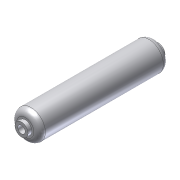
# Autodesk Inventor part: Pneuare Tank
Saved by Autodesk Inventor 2012 (Build 160160000, 160)
## iProperties
Created: 2013-02-02
Part Number: Pneuare Tank
Material: Polypropylene
Document SubType Name: Modeling
Designer: JesseK
Density: 0.899 g/cm^3
Mass: 311.75 g
Surface Area: 1100.4 cm^2
Volume: 346.774 cm^3
Author: JesseK
Autodesk Inventor part; units mm, degrees
ref_plane "YZ Plane" through (0, 0, 0) normal (1, 0, 0) x (0, 1, 0)
ref_plane "XZ Plane" through (0, 0, 0) normal (0, 1, 0) x (-1, 0, 0)
ref_plane "XY Plane" through (0, 0, 0) normal (0, 0, 1) x (1, 0, 0)
sketch "Sketch1" plane through (0, 0, 0) normal (0, 0, 1) x (1, 0, 0)
  circle A0 centre (0, 0) radius 31.75
  dimension "d0" = 63.5
  constraints: 1 centre point, 1 coincident
  measures "d0" diameter of A0
extrude "Extrusion1" add sketch "Sketch1" along normal blind 286.0294
sketch "Sketch2" plane through (0, 0, 286.0294) normal (0, 0, 1) x (1, 0, 0)
  circle A0 centre (0, 0) radius 31.75 projected
  circle A1 centre (0, 0) radius 14.5034
  dimension "d3" = 29.0068
  constraints: 1 centre point, 1 coincident
  measures "d3" diameter of A1
extrude "Extrusion2" add sketch "Sketch2" along normal blind 8.3566 contours A1
sketch "Sketch3" plane through (0, 0, 0) normal (0, 0, -1) x (-1, 0, 0)
  circle A0 centre (0, 0) radius 31.75 projected
  circle A1 centre (0, 0) radius 14.5034
  dimension "d6" = 29.0068
  constraints: 1 centre point, 1 coincident
  measures "d6" diameter of A1
extrude "Extrusion3" add sketch "Sketch3" along normal blind 8.3566 contours A1
fillet "Fillet1" radius 12.7 2 edges at (-31.75, 0, 0) (-31.75, 0, 286.0294)
shell "Shell1" thickness 6.35 removed faces 2 at (0.6824, -3.9787, -8.3566) at (-0.6824, -3.9787, 294.386)
body "Solid1"
